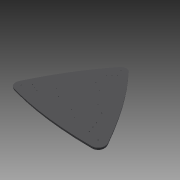
# Autodesk Inventor part: BOT PLATE
Saved by Autodesk Inventor 2013 (Build 170138000, 138)
## iProperties
Created: 2013-12-04
Part Number: BOT PLATE
Material: Generic
Document SubType Name: Modeling
Designer: employee
Density: 1 g/cm^3
Author: employee
Autodesk Inventor part; units mm, degrees
ref_plane "YZ Plane" through (0, 0, 0) normal (1, 0, 0) x (0, 1, 0)
ref_plane "XZ Plane" through (0, 0, 0) normal (0, 1, 0) x (-1, 0, 0)
ref_plane "XY Plane" through (0, 0, 0) normal (0, 0, 1) x (1, 0, 0)
sketch "Sketch1" plane through (0, 0, 0) normal (0, 0, 1) x (1, 0, 0)
  line L0 (0, -144.3376) -> (-125, 72.1688) construction
  line L1 (-125, 72.1688) -> (125, 72.1688) construction
  line L2 (125, 72.1688) -> (0, -144.3376) construction
  line L3 (0, 173.2051) -> (150, -86.6025) construction
  line L4 (150, -86.6025) -> (-150, -86.6025) construction
  line L5 (-150, -86.6025) -> (0, 173.2051) construction
  circle A0 centre (-150, -86.6025) radius 1.5875
  circle A1 centre (150, -86.6025) radius 1.5875
  circle A2 centre (0, 173.2051) radius 1.5875
  circle A3 centre (-125, 72.1688) radius 4.25
  circle A4 centre (125, 72.1688) radius 4.25
  circle A5 centre (0, -144.3376) radius 4.25
  circle A6 centre (-150, -86.6025) radius 25 construction
  line L6 (-250.0151, -144.3463) -> (0, 288.6926) construction
  line L7 (0, 288.6926) -> (250.0151, -144.3463) construction
  line L8 (250.0151, -144.3463) -> (-250.0151, -144.3463) construction
  arc A7 (-225.5835, -102.5089) -> (-201.5671, -144.1066) centre (-197.7721, -114.1838) ccw
  circle A8 centre (-125, 72.1688) radius 12.5 construction
  arc A9 (24.0164, 246.6155) -> (-24.0164, 246.6155) centre (0, 228.3676) ccw
  arc A10 (201.5671, -144.1066) -> (225.5835, -102.5089) centre (197.7721, -114.1838) ccw
  arc A11 (-24.0164, 246.6155) -> (-225.5835, -102.5089) centre (1251.5935, -722.6079) ccw
  arc A12 (225.5835, -102.5089) -> (24.0164, 246.6155) centre (-1251.5935, -722.6079) ccw
  arc A13 (-201.5671, -144.1066) -> (201.5671, -144.1066) centre (0, 1445.2157) ccw
  circle A14 centre (0, 228.3676) radius 1.5875
  circle A15 centre (-197.7721, -114.1838) radius 1.5875
  circle A16 centre (197.7721, -114.1838) radius 1.5875
  point P0 (0, 0)
  point P1 (0, 0)
  point P2 (0, 0)
  point P3 (0, 0)
  dimension "d0" = 300
  dimension "d1" = 250
  dimension "d2" = 3.175
  dimension "d3" = 8.5
  dimension "d4" = 50
  dimension "d5" = 60.325
  dimension "d6" = 25
  dimension "d9" = 3.175
  constraints: 18 end point, 17 centre point, 14 coincident, 14 tangent, 12 point on circle, 10 equal radius, 3 horizontal, 21 other
  measures "d0" distance of L3.end L4.end
  measures "d1" distance of L0.end L1.end
  measures "d2" diameter of A0
  measures "d3" diameter of A5
  measures "d4" diameter of A6
  measures "d5" diameter of A7
  measures "d6" diameter of A8
  measures "d9" diameter of A15
extrude "Extrusion2" add sketch "Sketch1" along normal blind 12.5 contours A3 | A4 | A5 | A11 A9 A12 A10 A13 A7
sketch "Sketch8" plane through (0, 0, 12.5) normal (0, 0, 1) x (1, 0, 0)
  circle A0 centre (0, 173.2051) radius 1.5875 projected
  line L0 (15.5, 157.7051) -> (-15.5, 157.7051) construction
  line L1 (-15.5, 157.7051) -> (-15.5, 188.7051) construction
  line L2 (-15.5, 188.7051) -> (15.5, 188.7051) construction
  line L3 (15.5, 188.7051) -> (15.5, 157.7051) construction
  circle A1 centre (-15.5, 157.7051) radius 1.6
  circle A2 centre (15.5, 188.7051) radius 1.6
  point P0 (0, 0)
  dimension "d34" = 3.2
  dimension "d36" = 31
  constraints: 8 end point, 3 coincident, 2 centre point, 1 equal radius, 1 horizontal, 9 other
  measures "d34" diameter of A2
  measures "d36" distance of L1.end L2.end
extrude "Extrusion9" cut sketch "Sketch8" against normal through all contours A1 | A2
pattern_circular "Circular Pattern1" count 3 over 360 about axis through (0, 0, -10) along (0, 0, 1) of "Extrusion9"
sketch "Sketch9" plane through (0, 0, 0) normal (0, 0, -1) x (-1, 0, 0)
  circle A0 centre (43.0398, -61.7471) radius 1.621 projected
  circle A1 centre (11.3411, 93.1567) radius 1.621 projected
  circle A2 centre (-31.9602, 68.1567) radius 1.621 projected
  circle A3 centre (86.3411, -36.7471) radius 1.621 projected
  line L0 (-76.356, 80.0525) -> (31.144, -106.143) projected
  line L1 (31.144, -106.143) -> (130.7369, -48.643) projected
  line L2 (130.7369, -48.643) -> (23.2369, 137.5525) projected
  line L3 (23.2369, 137.5525) -> (-76.356, 80.0525) projected
  line L4 (-51.5025, -76.895) -> (-72.9929, -89.3025) projected
  arc A4 (-79.8231, -87.4724) -> (-72.9929, -89.3025) centre (-75.4929, -84.9724) ccw projected
  line L5 (-79.8231, -87.4724) -> (-115.6621, -25.3974) projected
  arc A5 (-113.8319, -18.5673) -> (-115.6621, -25.3974) centre (-111.3319, -22.8974) ccw projected
  line L6 (-113.8319, -18.5673) -> (-92.3415, -6.1598) projected
  arc A6 (-85.5114, -7.9899) -> (-92.3415, -6.1598) centre (-89.8415, -10.4899) ccw projected
  line L7 (-85.5114, -7.9899) -> (-49.6724, -70.0649) projected
  arc A7 (-51.5025, -76.895) -> (-49.6724, -70.0649) centre (-54.0025, -72.5649) ccw projected
  circle A8 centre (-41.0253, -76.0422) radius 1.5 projected
  circle A9 centre (-78.9702, -97.9497) radius 1.5 projected
  circle A10 centre (-86.3643, 2.4873) radius 1.5 projected
  arc A11 (-125.8092, -16.8221) -> (-126.9072, -20.9202) centre (-124.3092, -19.4202) ccw projected
  line L8 (-126.9072, -20.9202) -> (-81.5682, -99.4497) projected
  arc A12 (-81.5682, -99.4497) -> (-77.4702, -100.5477) centre (-78.9702, -97.9497) ccw projected
  line L9 (-77.4702, -100.5477) -> (-39.5253, -78.6402) projected
  arc A13 (-39.5253, -78.6402) -> (-38.4272, -74.5422) centre (-41.0253, -76.0422) ccw projected
  line L10 (-38.4272, -74.5422) -> (-83.7662, 3.9873) projected
  arc A14 (-83.7662, 3.9873) -> (-87.8643, 5.0854) centre (-86.3643, 2.4873) ccw projected
  line L11 (-87.8643, 5.0854) -> (-125.8092, -16.8221) projected
  circle A15 centre (-124.3092, -19.4202) radius 1.5 projected
  point P0 (0, 0)
extrude "Extrusion10" cut sketch "Sketch9" against normal through all contours A0 | A1 | A2 | A3 | A8 | A9 | A10 | A15
fillet "Fillet2" radius 6.35 6 edges at (0, 258.5301, 0) (135.8253, 78.4188, 0) (223.8936, -129.265, 0) (0, -156.8376, 0) (-223.8936, -129.265, 0) (-135.8253, 78.4188, 0)
sketch "Sketch2" plane through (0, 0, 12.5) normal (0, 0, 1) x (1, 0, 0)
  circle A0 centre (0, 0) radius 105
  dimension "d12" = 210
  constraints: 1 centre point, 1 coincident
  measures "d12" diameter of A0
sketch "Sketch3" plane through (0, 0, 10.595) normal (0, 0, 1) x (1, 0, 0)
  circle A0 centre (0, 0) radius 105 projected
  line L0 (-31.25, 100.2419) -> (-31.25, 30)
  line L1 (-31.25, 30) -> (31.25, 30)
  line L2 (31.25, 30) -> (31.25, 100.2419)
  line L3 (0, 30) -> (0, 105) construction
  dimension "d16" = 75
  dimension "d18" = 62.5
  constraints: 8 end point, 3 point on circle, 2 parallel, 1 midpoint, 1 perpendicular, 1 vertical, 1 vertical alignment
  measures "d16" distance of L3.start L3.end
  measures "d18" distance between parallel lines of L2 L0
sketch "Sketch4" plane through (0, 0, 12.5) normal (0, 0, 1) x (1, 0, 0)
  circle A0 centre (0, 0) radius 105 projected
  circle A1 centre (0, 105) radius 12.5
  dimension "d21" = 25
  constraints: 2 vertical alignment, 1 centre point, 1 other
  measures "d21" diameter of A1
sketch "Sketch5" plane through (0, 0, 12.5) normal (0, 0, 1) x (1, 0, 0)
  arc A0 (24.0164, 246.6155) -> (-24.0164, 246.6155) centre (0, 228.3676) ccw projected
  arc A1 (201.5671, -144.1066) -> (225.5835, -102.5089) centre (197.7721, -114.1838) ccw projected
  circle A2 centre (0, 228.3676) radius 1.5875 projected
  circle A3 centre (-197.7721, -114.1838) radius 1.5875 projected
  circle A4 centre (197.7721, -114.1838) radius 1.5875 projected
  circle A5 centre (0, 228.3676) radius 30.1625
  circle A6 centre (197.7721, -114.1838) radius 30.1625
  circle A7 centre (-197.7721, -114.1838) radius 30.1625
  constraints: 3 centre point, 3 coincident, 3 equal radius
sketch "Sketch6" plane through (-193.442, -111.6838, 571.3) normal (0, 0, 1) x (1, 0, 0)
  circle A0 centre (0, 0) radius 1.5875 projected
  circle A1 centre (0, 0) radius 30.1625 projected
  arc A2 (205.9198, 215.9397) -> (180.9642, 215.9397) centre (193.442, 216.6838) ccw projected
  arc A3 (180.9642, 215.9397) -> (205.9198, 215.9397) centre (193.442, 111.6838) ccw projected
  circle A4 centre (193.442, -32.6538) radius 4.25 projected
  circle A5 centre (318.442, 183.8526) radius 4.25 projected
  circle A6 centre (68.442, 183.8526) radius 4.25 projected
  circle A7 centre (193.442, 284.8889) radius 1.5875 projected
  circle A8 centre (343.442, 25.0812) radius 1.5875 projected
  circle A9 centre (43.442, 25.0812) radius 1.5875 projected
  arc A10 (-4.6471, -29.8024) -> (-28.1332, 10.8766) centre (0, 0) ccw projected
  arc A11 (-4.6471, -29.8024) -> (391.5311, -29.8024) centre (193.442, 1240.5571) ccw projected
  arc A12 (415.0172, 10.8766) -> (391.5311, -29.8024) centre (386.884, 0) ccw projected
  arc A13 (415.0172, 10.8766) -> (216.928, 353.9771) centre (-784.1909, -452.7528) ccw projected
  arc A14 (169.956, 353.9771) -> (216.928, 353.9771) centre (193.442, 335.0514) ccw projected
  arc A15 (169.956, 353.9771) -> (-28.1332, 10.8766) centre (1171.0749, -452.7528) ccw projected
  circle A16 centre (193.442, 335.0514) radius 1.5875 projected
  circle A17 centre (193.442, 335.0514) radius 30.1625 projected
  circle A18 centre (386.884, 0) radius 1.5875 projected
  circle A19 centre (386.884, 0) radius 30.1625 projected
sketch "Sketch7" plane through (-193.442, -111.6838, -89.1) normal (0, 0, -1) x (-1, 0, 0)
  circle A0 centre (0, 0) radius 30.1625 projected
  circle A1 centre (-68.442, 183.8526) radius 4.25 projected
  circle A2 centre (-318.442, 183.8526) radius 4.25 projected
  circle A3 centre (-193.442, -32.6538) radius 4.25 projected
  circle A4 centre (-43.442, 25.0812) radius 1.5875 projected
  circle A5 centre (-343.442, 25.0812) radius 1.5875 projected
  circle A6 centre (-193.442, 284.8889) radius 1.5875 projected
  circle A7 centre (-386.884, 0) radius 1.5875 projected
  circle A8 centre (-193.442, 335.0514) radius 1.5875 projected
  circle A9 centre (0, 0) radius 1.5875 projected
  arc A10 (-169.956, 353.9771) -> (-216.928, 353.9771) centre (-193.442, 335.0514) ccw projected
  arc A11 (28.1332, 10.8766) -> (-169.956, 353.9771) centre (-1171.0749, -452.7528) ccw projected
  arc A12 (-391.5311, -29.8024) -> (4.6471, -29.8024) centre (-193.442, 1240.5571) ccw projected
  arc A13 (-415.0172, 10.8766) -> (-391.5311, -29.8024) centre (-386.884, 0) ccw projected
  arc A14 (-216.928, 353.9771) -> (-415.0172, 10.8766) centre (784.1909, -452.7528) ccw projected
  arc A15 (4.6471, -29.8024) -> (28.1332, 10.8766) centre (0, 0) ccw projected
  point P0 (-193.442, 111.6838)
body "Solid2"
